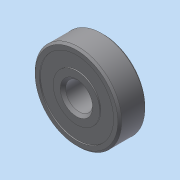
# Autodesk Inventor part: 625 2RS Bearing
Saved by Autodesk Inventor 2013 (Build 170138000, 138)
## iProperties
Created: 2013-12-11
Part Number: 625 2RS Bearing
Material: Generic
Document SubType Name: Modeling
Designer: Work
Density: 1 g/cm^3
Author: Work
Autodesk Inventor part; units mm, degrees
ref_plane "YZ Plane" through (0, 0, 0) normal (1, 0, 0) x (0, 1, 0)
ref_plane "XZ Plane" through (0, 0, 0) normal (0, 1, 0) x (-1, 0, 0)
ref_plane "XY Plane" through (0, 0, 0) normal (0, 0, 1) x (1, 0, 0)
sketch "Sketch1" plane through (0, 0, 0) normal (0, 0, 1) x (1, 0, 0)
  line L0 (0, 0) -> (0, 2.5)
  line L1 (-2.5, 0) -> (-2.5, 2)
  line L2 (-2.5, 2) -> (-3, 2.5)
  line L3 (-3, 2.5) -> (-4.3, 2.5)
  line L4 (-4.3, 2.5) -> (-4.3, 2.3)
  line L5 (-4.3, 2.3) -> (-6.85, 2.3)
  line L6 (-6.85, 2.3) -> (-6.85, 2.5)
  line L7 (-6.85, 2.5) -> (-7.6465, 2.5)
  line L8 (-7.6465, 2.5) -> (-8, 2.1465)
  line L9 (-8, 2.1465) -> (-8, 0)
  line L10 (-8, 0) -> (-2.5, 0)
  dimension "d9" = 2.5
  dimension "d19" = 2.5
  dimension "d20" = 0.2
  dimension "d21" = 5
  dimension "d22" = 6
  dimension "d23" = 8.6
  dimension "d24" = 13.7
  dimension "d26" = 16
  dimension "d27" = 135
  dimension "d29" = 0.5
  dimension "d30" = 15.293
  constraints: 22 end point, 5 parallel, 3 perpendicular, 2 collinear, 1 point on line, 1 vertical
  measures "d9" distance of L0.start L0.end
  measures "d19" distance between parallel lines of L10 L3
  measures "d20" distance between parallel lines of L3 L5
  measures "d21" diameter of L1 L0
  measures "d22" diameter of L2.end L0
  measures "d23" diameter of L4 L0
  measures "d24" diameter of L6 L0
  measures "d26" diameter of L9 L0
  measures "d27" angle of L1 L2
  measures "d29" horizontal distance of L2.end L1.end
  measures "d30" diameter of L7.end L0
revolve "Revolution1" add sketch "Sketch1" angle 360 about axis through (0, 0, 0) along (0, 1, 0)
mirror "Mirror1" about plane through (-5.25, 0, 0) normal (0, -1, 0) of "Revolution1"
equation "\"d19\" = d9"
body "Solid1"
